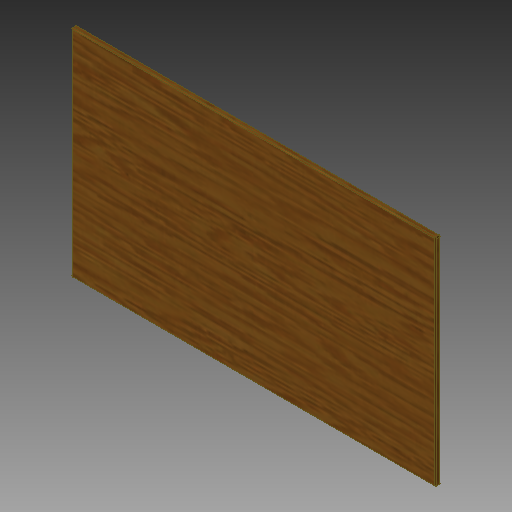
# Autodesk Inventor part: 2124_Plywood Frame Top_V1
Saved by Autodesk Inventor 2020 (Build 240168000, 168)
## iProperties
Created: 2019-10-13
Part Number: 2124_Plywood Frame Top_V1
Material: Plywood, Finish
Document SubType Name: Modeling
Designer: RFLab
Density: 0.552 g/cm^3
Appearance: Plywood - New
Mass: 1601.43 g
Surface Area: 5994.33 cm^2
Volume: 2901.15 cm^3
Author: RFLab
Autodesk Inventor part; units mm, degrees
ref_plane "YZ Plane" through (0, 0, 0) normal (1, 0, 0) x (0, 1, 0)
ref_plane "XZ Plane" through (0, 0, 0) normal (0, 1, 0) x (-1, 0, 0)
ref_plane "XY Plane" through (0, 0, 0) normal (0, 0, 1) x (1, 0, 0)
sketch "Sketch1" plane through (0, 0, 0) normal (0, 0, 1) x (1, 0, 0)
  line L0 (-350, -207.5) -> (350, -207.5)
  line L1 (350, -207.5) -> (350, 207.5)
  line L2 (350, 207.5) -> (-350, 207.5)
  line L3 (-350, 207.5) -> (-350, -207.5)
  line L4 (-350, -207.5) -> (350, 207.5) construction
  line L5 (350, -207.5) -> (-350, 207.5) construction
  point P0 (0, 0)
  dimension "d0" = 700
  dimension "d1" = 415
  constraints: 12 end point, 2 midpoint, 2 parallel, 1 horizontal, 1 perpendicular
  measures "d0" distance of L2.end L1.end
  measures "d1" distance of L1.end L0.end
extrude "Extrusion1" add sketch "Sketch1" along normal blind 10
fillet "Fillet1" radius 2 12 edges at (0, -207.5, 10) (0, -207.5, 0) (350, -207.5, 5) (350, 0, 10) (350, 0, 0) (350, 207.5, 5) (0, 207.5, 10) (0, 207.5, 0) (-350, 207.5, 5) (-350, 0, 10) (-350, -207.5, 5) (-350, 0, 0)
body "Solid1"
